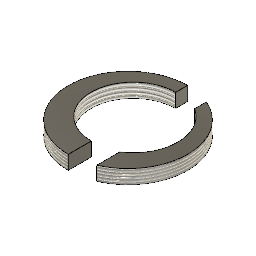
Buoyani-3D-v0 (Autodesk Fusion 360 design; units mm, degrees)
Autodesk Fusion 360 part; units mm, degrees
note: some values were not read from the file. Chosen so that the rebuilt part matches the saved one: which bodies a step acts on; which face or edge a step refers to; how an offset face is resized.
cylinder "CylinderPrimitive1" add diameter 252.116 height 30 placed x (1, 0, 0) y (0, 1, 0) z (0, 0, 1) at (0, 0, 0) makes body 1
hole "Hole1" at (-0.7878, 11.9201, 30) direction (0, 0, -1) diameter 180 depth 40 tip angle 118 bodies 1
cylinder "CylinderPrimitive2" cut diameter 427.551 height 50 placed x (0, 0, -1) y (0, 1, 0) z (1, 0, 0) at (0, 0, 0) bodies 1 makes body 2 at (85.6533, 92.4885, 10)
thread "Thread1" "ISO Metric profile 200.0 M200x8 6H" major diameter 200.8149 minor diameter 191.8397 pitch 8 angle 60 resizes the face on face at (-84.2698, -21.7067, 10) on bodies 1
thread "Thread2" "ISO Metric profile 255.0 M255x6 6g" major diameter 254.62 minor diameter 247.6983 pitch 6 angle 60 resizes the face on face at (85.6533, 92.4885, 10) on bodies 2
thread "Thread3" "ISO Metric profile 195.0 M195x6 6H" major diameter 195.6455 minor diameter 188.9048 pitch 6 angle 60 resizes the face on face at (57.1371, -56.9616, 10) on bodies 2
thread "Thread4" "ISO Metric profile 255.0 M255x6 6g" major diameter 254.62 minor diameter 247.6983 pitch 6 angle 60 resizes the face on face at (-105.892, 68.3923, 20) on bodies 1
thread "Thread5" "ISO Metric profile 185.0 M185x6 6H" major diameter 185.6455 minor diameter 178.9048 pitch 6 angle 60 resizes the face on face at (-69.9442, -54.5481, 20) on bodies 1
